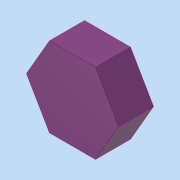
# Autodesk Inventor part: NarrowHexNutCaps
Saved by Autodesk Inventor 2017 (Build 210142000, 142)
## iProperties
Created: 2018-04-10
Part Number: NarrowHexNutCaps
Material: ABS Plastic
Document SubType Name: Modeling
Designer: Derek Wider
Density: 1.06 g/cm^3
Appearance: Smooth - Purple
Author: Derek Wider
Autodesk Inventor part; units mm, degrees
ref_plane "YZ Plane" through (0, 0, 0) normal (1, 0, 0) x (0, 1, 0)
ref_plane "XZ Plane" through (0, 0, 0) normal (0, 1, 0) x (-1, 0, 0)
ref_plane "XY Plane" through (0, 0, 0) normal (0, 0, 1) x (1, 0, 0)
sketch "Sketch1" plane through (0, 0, 0) normal (0, 0, 1) x (1, 0, 0)
  line L0 (-3.8128, 0) -> (-1.9064, 3.302)
  line L1 (-1.9064, 3.302) -> (1.9064, 3.302)
  line L2 (1.9064, 3.302) -> (3.8128, 0)
  line L3 (3.8128, 0) -> (1.9064, -3.302)
  line L4 (1.9064, -3.302) -> (-1.9064, -3.302)
  line L5 (-1.9064, -3.302) -> (-3.8128, 0)
  line L6 (-5.4993, 0) -> (-2.7496, 4.7625)
  line L7 (-2.7496, 4.7625) -> (2.7496, 4.7625)
  line L8 (2.7496, 4.7625) -> (5.4993, 0)
  line L9 (5.4993, 0) -> (2.7496, -4.7625)
  line L10 (2.7496, -4.7625) -> (-2.7496, -4.7625)
  line L11 (-2.7496, -4.7625) -> (-5.4993, 0)
  point P0 (0, 0)
  point P1 (0, 0)
  point P2 (0, 0)
  dimension "d0" = 6.604
  dimension "d1" = 9.525
  constraints: 24 end point, 2 coincident, 26 other
  measures "d0" distance between parallel lines of L4 L1
  measures "d1" distance between parallel lines of L10 L7
extrude "Extrusion1" add sketch "Sketch1" along normal blind 4.191 contours L0 L1 L2 L3 L4 L5 | L6 L7 L8 L9 L10 L11
extrude "Extrusion2" cut sketch "Sketch1" along normal blind 2.794 contours L0 L1 L2 L3 L4 L5
body "Solid1"
